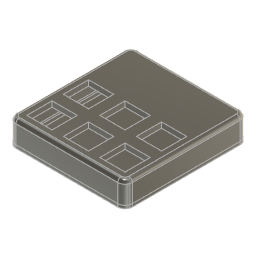
w3by2 (Autodesk Fusion 360 design; units mm, degrees)
Autodesk Fusion 360 part; units mm, degrees
sketch "Sketch1" plane through (0, 0, 0) normal (0, 0, 1) x (1, 0, 0)
  line L0 (4, 0) -> (59.8, 0)
  line L1 (63.8, 4) -> (63.8, 63.0607)
  line L2 (59.8, 67.0607) -> (4, 67.0607)
  line L3 (0, 63.0607) -> (0, 4)
  line L4 (5, 5) -> (18.8, 5)
  line L5 (18.8, 5) -> (18.8, 18.8)
  line L6 (18.8, 18.8) -> (5, 18.8)
  line L7 (5, 18.8) -> (5, 5)
  line L8 (38.8, 18.8) -> (25, 18.8)
  line L9 (25, 18.8) -> (25, 5)
  line L10 (38.8, 5) -> (38.8, 18.8)
  line L11 (25, 5) -> (38.8, 5)
  line L12 (58.8, 18.8) -> (45, 18.8)
  line L13 (45, 18.8) -> (45, 5)
  line L14 (58.8, 5) -> (58.8, 18.8)
  line L15 (45, 5) -> (58.8, 5)
  line L16 (18.8, 38.8) -> (5, 38.8)
  line L17 (5, 38.8) -> (5, 25)
  line L18 (18.8, 25) -> (18.8, 38.8)
  line L19 (5, 25) -> (18.8, 25)
  line L20 (38.8, 38.8) -> (25, 38.8)
  line L21 (25, 38.8) -> (25, 25)
  line L22 (38.8, 25) -> (38.8, 38.8)
  line L23 (25, 25) -> (38.8, 25)
  line L24 (58.8, 38.8) -> (45, 38.8)
  line L25 (45, 38.8) -> (45, 25)
  line L26 (58.8, 25) -> (58.8, 38.8)
  line L27 (45, 25) -> (58.8, 25)
  line L28 (2, 61.5603) -> (35.81, 61.5603)
  line L29 (35.81, 61.5603) -> (35.81, 43.3603)
  line L30 (35.81, 43.3603) -> (2, 43.3603)
  line L31 (35.3999, 45.3501) -> (6, 45.3501)
  line L32 (6, 59.5501) -> (35.3999, 59.5501)
  line L33 (37.3999, 63.6019) -> (37.3999, 41.3501)
  line L34 (37.3999, 41.3501) -> (31.9039, 41.3501)
  line L35 (31.9039, 43.3603) -> (31.9039, 41.3501)
  line L36 (31.8901, 61.5603) -> (31.8901, 63.6019)
  line L37 (33.4999, 47.2503) -> (7.9001, 47.2503)
  line L38 (7.9001, 57.65) -> (33.4999, 57.65)
  line L39 (33.4999, 57.65) -> (35.81, 57.65)
  line L40 (7.9001, 57.65) -> (2, 57.6034)
  line L41 (7.9001, 47.2503) -> (2, 47.3114)
  line L42 (33.4999, 47.2503) -> (35.81, 47.2503)
  line L43 (6, 59.5501) -> (2, 59.5501)
  line L44 (35.3999, 59.5501) -> (35.81, 59.5501)
  line L45 (6, 45.3501) -> (2, 45.3501)
  line L46 (35.3999, 45.3501) -> (35.81, 45.3501)
  arc A0 (0, 4) -> (4, 0) centre (4, 4) ccw
  arc A1 (59.8, 0) -> (63.8, 4) centre (59.8, 4) ccw
  arc A2 (63.8, 63.0607) -> (59.8, 67.0607) centre (59.8, 63.0607) ccw
  arc A3 (4, 67.0607) -> (0, 63.0607) centre (4, 63.0607) ccw
  line L47 (4, 2) -> (59.8, 2)
  arc A4 (59.8, 2) -> (61.8, 4) centre (59.8, 4) ccw
  line L48 (61.8, 4) -> (61.8, 63.0607)
  arc A5 (61.8, 63.0607) -> (59.8, 65.0607) centre (59.8, 63.0607) ccw
  line L49 (59.8, 65.0607) -> (4, 65.0607)
  arc A6 (4, 65.0607) -> (2, 63.0607) centre (4, 63.0607) ccw
  line L50 (2, 63.0607) -> (2, 4)
  arc A7 (2, 4) -> (4, 2) centre (4, 4) ccw
  line L51 (2, 63.6019) -> (2.0746, 63.6019)
  line L52 (31.8901, 63.6019) -> (37.3999, 63.6019)
  dimension "d1" = 13.8
  dimension "d2" = 13.8
  dimension "d6" = 20
  dimension "d7" = 20
  dimension "d9" = 5
  dimension "d10" = 5
  dimension "d11" = 5
  dimension "d13" = -2
  dimension "d90" = 33.81
  dimension "d91" = 18.2
  dimension "d108" = 4
  dimension "d122" = 67.0607
  constraint horizontal L0
  constraint vertical L1
  constraint horizontal L2
  constraint vertical L3
  constraint horizontal L4
  constraint vertical L5
  constraint horizontal L6
  constraint vertical L7
  constraint horizontal L28
  constraint vertical L29
  constraint horizontal L30
  constraint coincident L30 L35.start
  constraint perpendicular L34 L35
  constraint coincident L28 L36.start
  constraint coincident L36.end L51
  constraint perpendicular L36 L51
  constraint coincident L29 L39.end
  constraint perpendicular L29 L39
  constraint coincident L29 L42.end
  constraint perpendicular L29 L42
  constraint horizontal L43
  constraint coincident L29 L44.end
  constraint perpendicular L29 L44
  constraint horizontal L45
  constraint coincident L45.end L50
  constraint coincident L29 L46.end
  constraint perpendicular L29 L46
  constraint tangent L0 A0
  constraint tangent L3 A0
  constraint tangent L0 A1
  constraint tangent L1 A1
  constraint equal A0 A1
  constraint tangent L1 A2
  constraint tangent L2 A2
  constraint equal A0 A2
  constraint tangent L2 A3
  constraint tangent L3 A3
  constraint equal A0 A3
  constraint coincident origin L0
  constraint coincident origin L3
  constraint parallel L30 L37
  constraint parallel L28 L38
  constraint parallel L30 L31
  constraint parallel L28 L32
  constraint parallel L28 L51
  constraint parallel L29 L33
  constraint parallel L30 L34
  constraint coincident L41.end L50
  constraint coincident L50 L40.end
  constraint coincident L28.start L50
  constraint coincident L30.end L50
  constraint coincident L43.end L50
  constraint coincident A6 L51.end
  constraint collinear L51 L52
  measures "d1" distance of L4.start L4.end
  measures "d2" distance of L4.start L6.end
  measures "d9" distance of L0 L4
  measures "d10" distance of L3 L7
  measures "d11" distance of L1 L14
  measures "d90" distance of L28.start L28.end
  measures "d91" distance of L28.start L30.end
  measures "d108" radius of A0
  measures "d122" distance of L0 L2
extrude "Extrude1" add sketch "Sketch1" along normal blind 3 contours L0 L1 L2 L3 A0 A1 A2 A3 | L28 L30 L33 L34 L35 L36 L47 A4 L48 A5 L49 A6 L50 A7 L52 | L28 L29 L32 L43 L44 L50 | L28 L29 L30 L33 L34 L35 L36 L52 | L29 L32 L38 L39 L40 L43 L44 L50 | L29 L37 L38 L39 L40 L41 L42 L50 | L29 L31 L37 L41 L42 L45 L46 L50 | L29 L30 L31 L45 L46 L50 makes body 1
extrude "Extrude6" add sketch "Sketch1" against normal blind 9 contours L0 L1 L2 L3 A0 A1 A2 A3 bodies 1
extrude "Extrude20" add sketch "Sketch1" against normal blind 3 contours L28 L29 L30 L33 L34 L35 L36 L52 bodies 1
extrude "Extrude21" add sketch "Sketch1" against normal blind 1.5 contours L29 L32 L38 L39 L40 L43 L44 L50 | L29 L31 L37 L41 L42 L45 L46 L50 bodies 1
sketch "Sketch9" plane through (2, 0, 0) normal (1, 0, 0) x (0, 1, 0)
  line L0 (4, -9) -> (63.0607, -9)
  line L1 (50.6154, -6) -> (54.6154, -6)
  arc A0 (54.6154, -6) -> (54.6154, -2) centre (54.6154, -4) ccw
  line L2 (54.6154, -2) -> (50.6154, -2)
  arc A1 (50.6154, -2) -> (50.6154, -6) centre (50.6154, -4) ccw
  line L3 (48.6154, -4) -> (56.6154, -4) construction
  line L4 (63.0607, 0) -> (4, 0)
  line L5 (4, 0) -> (4, -9)
  line L6 (63.0607, -9) -> (63.0607, 0)
  line L7 (45.3501, 0) -> (4, 0)
  line L8 (47.3114, 0) -> (47.3114, -1.5)
  line L9 (47.3114, -1.5) -> (45.3501, -1.5)
  line L10 (45.3501, -1.5) -> (45.3501, 0)
  line L11 (63.0607, 0) -> (59.5501, 0)
  line L12 (59.5501, 0) -> (59.5501, -1.5)
  line L13 (59.5501, -1.5) -> (57.6034, -1.5)
  line L14 (57.6034, -1.5) -> (57.6034, 0)
  line L15 (57.6034, 0) -> (47.3114, 0)
  dimension "d100" = 4
  dimension "d104" = 2
  constraint tangent L1 A0
  constraint tangent A0 L2
  constraint parallel L1 L2
  constraint tangent L2 A1
  constraint tangent L1 A1
  constraint midpoint A1 L3.start
  constraint midpoint A0 L3.end
  measures "d100" diameter of A0
  measures "d104" distance of L2 L4
extrude "Extrude22" cut sketch "Sketch9" against normal blind 8 contours L1 A0 L2 A1 bodies 1
sketch "Sketch10" plane through (0, 0, -9) normal (0, 0, -1) x (1, 0, 0)
  arc A0 (4, -2) -> (2, -4) centre (4, -4) ccw
  line L0 (4, -2) -> (59.8, -2)
  arc A1 (61.8, -4) -> (59.8, -2) centre (59.8, -4) ccw
  line L1 (61.8, -4) -> (61.8, -63.0607)
  arc A2 (59.8, -65.0607) -> (61.8, -63.0607) centre (59.8, -63.0607) ccw
  line L2 (59.8, -65.0607) -> (4, -65.0607)
  arc A3 (2, -63.0607) -> (4, -65.0607) centre (4, -63.0607) ccw
  line L3 (2, -63.0607) -> (2, -4)
  arc A4 (0, -63.0607) -> (4, -67.0607) centre (4, -63.0607) ccw
  line L4 (4, -67.0607) -> (59.8, -67.0607)
  arc A5 (59.8, -67.0607) -> (63.8, -63.0607) centre (59.8, -63.0607) ccw
  line L5 (63.8, -63.0607) -> (63.8, -4)
  arc A6 (63.8, -4) -> (59.8, 0) centre (59.8, -4) ccw
  line L6 (59.8, 0) -> (4, 0)
  arc A7 (4, 0) -> (0, -4) centre (4, -4) ccw
  line L7 (0, -4) -> (0, -63.0607)
  arc A8 (61.6, -4) -> (59.8, -2.2) centre (59.8, -4) ccw
  line L8 (4, -2.2) -> (59.8, -2.2)
  arc A9 (4, -2.2) -> (2.2, -4) centre (4, -4) ccw
  line L9 (2.2, -63.0607) -> (2.2, -4)
  arc A10 (2.2, -63.0607) -> (4, -64.8607) centre (4, -63.0607) ccw
  line L10 (59.8, -64.8607) -> (4, -64.8607)
  arc A11 (59.8, -64.8607) -> (61.6, -63.0607) centre (59.8, -63.0607) ccw
  line L11 (61.6, -4) -> (61.6, -63.0607)
  arc A12 (60.6, -4) -> (59.8, -3.2) centre (59.8, -4) ccw
  line L12 (4, -3.2) -> (59.8, -3.2)
  arc A13 (4, -3.2) -> (3.2, -4) centre (4, -4) ccw
  line L13 (3.2, -63.0607) -> (3.2, -4)
  arc A14 (3.2, -63.0607) -> (4, -63.8607) centre (4, -63.0607) ccw
  line L14 (59.8, -63.8607) -> (4, -63.8607)
  arc A15 (59.8, -63.8607) -> (60.6, -63.0607) centre (59.8, -63.0607) ccw
  line L15 (60.6, -4) -> (60.6, -63.0607)
  line L16 (33.3999, -49.0564) -> (37.3999, -49.0564)
  line L17 (37.3999, -49.0564) -> (37.3999, -56.0564)
  line L18 (37.3999, -56.0564) -> (33.3999, -56.0564)
  line L19 (33.3999, -56.0564) -> (33.3999, -49.0564)
  line L20 (35.81, -61.5603) -> (35.81, -43.3603)
  line L21 (37.3999, -63.6019) -> (37.3999, -41.3501)
  line L22 (33.4999, -57.65) -> (35.81, -57.65)
  line L23 (2, -61.5603) -> (35.81, -61.5603)
  dimension "d109" = 0.2
  dimension "d110" = 1.2
  dimension "d117" = 7
  dimension "d118" = 4
  dimension "d119" = 5.5039
  constraint horizontal L16
  constraint vertical L17
  constraint horizontal L18
  constraint vertical L19
  constraint coincident L17.end L21
  measures "d117" distance of L16 L18
  measures "d118" distance of L17 L19
  measures "d119" distance of L18 L23
extrude "Extrude23" add sketch "Sketch10" along normal blind 1.6 separate body contours A0 L0 A1 L1 A2 L2 A3 L3 | A4 L4 A5 L5 A6 L6 A7 L7 | A8 L8 A9 L9 A10 L10 A11 L11 | A12 L12 A13 L13 A14 L14 A15 L15 | L16 L18 L19 L20 | L16 L17 L18 L20 L21 makes body 2
extrude "Extrude24" add sketch "Sketch10" against normal blind 2 contours A8 L8 A9 L9 A10 L10 A11 L11 bodies 2
fillet "Fillet6" radius 2 8 edges at (0, 33.5303, 3) (1.1716, 1.1716, 3) (31.9, 0, 3) (62.6284, 1.1716, 3) (63.8, 33.5303, 3) (62.6284, 65.8891, 3) (31.9, 67.0607, 3) (1.1716, 65.8891, 3) on bodies 1
extrude "Extrude25" add sketch "Sketch10" against normal up to surface (5.8 mm away) contours L16 L18 L19 L20 | L16 L17 L18 L20 L21 bodies 2
fillet "Fillet8" radius 1 6 edges at (31.9039, 41.3501, -1.5) (31.9039, 43.3603, -1.5) (37.3999, 41.3501, -1.5) (37.3999, 63.6019, -1.5) (31.8901, 63.6019, -1.5) (31.8901, 61.5603, -1.5) on bodies 1
equation "d1 = keyWidth"
equation "d2 = keyWidth"
equation "keyWidth = 13.8 mm"
equation "d6 = keySpacing"
equation "d7 = keySpacing"
equation "keySpacing = 20 mm"
equation "d10 = d9"
equation "d11 = d10"
equation "d90 = PromicroLength + 0.2 mm"
equation "PromicroLength = 33.61 mm"
named bodies: "switch holder", "cover"
